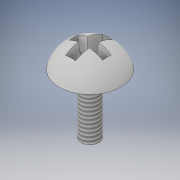
# Autodesk Inventor part: tiny screw
Saved by Autodesk Inventor 2017.1 (Build 211199000, 199)
## iProperties
Created: 2017-04-20
Part Number: tiny screw
Material: Generic
Document SubType Name: Modeling
Designer: 196918
Density: 1 g/cm^3
Appearance: Default
Author: 196918
Autodesk Inventor part; units mm, degrees
ref_plane "YZ Plane" through (0, 0, 0) normal (1, 0, 0) x (0, 1, 0)
ref_plane "XZ Plane" through (0, 0, 0) normal (0, 1, 0) x (-1, 0, 0)
ref_plane "XY Plane" through (0, 0, 0) normal (0, 0, 1) x (1, 0, 0)
sketch "Sketch1" plane through (0, 0, 0) normal (0, 1, 0) x (-1, 0, 0)
  circle A0 centre (0, 0) radius 1.905
  dimension "d0" = 3.81
  constraints: 1 centre point, 1 coincident
  measures "d0" diameter of A0
extrude "Extrusion1" add sketch "Sketch1" along normal blind 12.7
thread "Thread1" size "8-32 UNC" class "2A" standard "ANSI Unified Screw Threads" full length
sketch "Sketch2" plane through (0, 12.7, 0) normal (0, 1, 0) x (1, 0, 0)
  circle A0 centre (0, 0) radius 6.61892
  constraints: 1 centre point, 1 coincident
extrude "Extrusion2" add sketch "Sketch2" along normal blind 5.08
fillet "Fillet1" radius 6.35 1 edges at (-6.6189, 17.78, 0)
sketch "Sketch3" plane through (0, 17.78, 0) normal (0, 1, 0) x (1, 0, 0)
  line L0 (-3.495957, -1.079634) -> (3.804424, -1.079634)
  line L1 (3.804424, -1.079634) -> (3.804424, 0.9254)
  line L2 (3.804424, 0.9254) -> (-3.495957, 0.9254)
  line L3 (-3.495957, 0.9254) -> (-3.495957, -1.079634)
  line L4 (-1.439512, -4.010068) -> (0.9254, -4.010068)
  line L5 (0.9254, -4.010068) -> (0.9254, 4.11289)
  line L6 (0.9254, 4.11289) -> (-1.439512, 4.11289)
  line L7 (-1.439512, 4.11289) -> (-1.439512, -4.010068)
  point P0 (0, 0)
  constraints: 16 end point, 4 parallel, 2 horizontal, 2 perpendicular
sketch "Sketch3 outline for Extrusion3" plane through (0, 17.78, 0) normal (0, 1, 0) x (1, 0, 0)
  line L0 (-1.439512, 0.9254) -> (-3.495957, 0.9254)
  line L1 (-3.495957, 0.9254) -> (-3.495957, -1.079634)
  line L2 (-3.495957, -1.079634) -> (-1.439512, -1.079634)
  line L3 (-1.439512, -1.079634) -> (-1.439512, -4.010068)
  line L4 (-1.439512, -4.010068) -> (0.9254, -4.010068)
  line L5 (0.9254, -4.010068) -> (0.9254, -1.079634)
  line L6 (0.9254, -1.079634) -> (3.804424, -1.079634)
  line L7 (3.804424, -1.079634) -> (3.804424, 0.9254)
  line L8 (3.804424, 0.9254) -> (0.9254, 0.9254)
  line L9 (0.9254, 0.9254) -> (0.9254, 4.11289)
  line L10 (0.9254, 4.11289) -> (-1.439512, 4.11289)
  line L11 (-1.439512, 4.11289) -> (-1.439512, 0.9254)
extrude "Extrusion3" cut sketch "Sketch3 outline for Extrusion3" against normal blind 3.4925 draft -5
body "Solid1"
